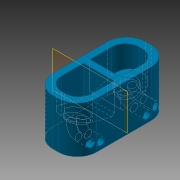
# Autodesk Inventor part: Line Tracker v3
Saved by Autodesk Inventor 2015 SP2 (Build 190223200, 223)
## iProperties
Created: 2015-04-19
Part Number: Line Tracker v3
Material: PLA Plastic
Document SubType Name: Modeling
Designer: Kyle
Density: 1 g/cm^3
Appearance: Carbon Fiber 1
Author: Kyle
Autodesk Inventor part; units mm, degrees
ref_plane "YZ Plane" through (0, 0, 0) normal (1, 0, 0) x (0, 1, 0)
ref_plane "XZ Plane" through (0, 0, 0) normal (0, 1, 0) x (-1, 0, 0)
sketch "Sketch1" plane through (0, 0, 0) normal (1, 0, 0) x (0, 1, 0)
  line L0 (0, 0) -> (0, 10.795)
  line L1 (0, 10.795) -> (10.795, 10.795)
  line L2 (10.795, 10.795) -> (10.795, 9.017)
  line L3 (10.795, 9.017) -> (5.8775, 9.017)
  line L4 (5.8775, 9.017) -> (3.81, 1.3008)
  line L5 (4.3488, 0.762) -> (10.795, 0.762)
  line L6 (10.795, 0.762) -> (10.795, 0)
  line L7 (0, 0) -> (10.795, 0) construction
  line L8 (3.81, 1.3008) -> (4.3488, 0.762)
  line L9 (0, 0) -> (0, -10.795)
  line L10 (0, -10.795) -> (10.795, -10.795)
  line L11 (10.795, -10.795) -> (10.795, -9.017)
  line L12 (10.795, -9.017) -> (5.8775, -9.017)
  line L13 (5.8775, -9.017) -> (3.81, -1.3008)
  line L14 (4.3488, -0.762) -> (10.795, -0.762)
  line L15 (10.795, -0.762) -> (10.795, 0)
  line L16 (3.81, -1.3008) -> (4.3488, -0.762)
  dimension "d0" = 10.795
  dimension "d1" = 105
  dimension "d8" = 0.762
  dimension "d33" = 3.81
  dimension "d34" = 10.795
  dimension "d35" = 0.762
  dimension "d36" = 1.778
  constraints: 34 end point, 7 symmetric about line, 4 perpendicular, 2 horizontal, 1 collinear, 1 vertical
  measures "d0" distance of L0.start L0.end
  measures "d1" angle of L4 L3
  measures "d8" distance of L5.end L6.end
  measures "d33" distance from line of L0 L4.end
  measures "d34" distance of L0.end L1.end
  measures "d35" distance of L4.end L5.start
  measures "d36" distance of L1.end L2.end
extrude "Extrusion1" add sketch "Sketch1" along normal mid plane 7.112
sketch "Sketch2" plane through (3.556, 0, 0) normal (1, 0, 0) x (0, 0, -1)
  line L0 (-10.795, 10.795) -> (10.795, 10.795)
  line L1 (10.795, 10.795) -> (10.795, 0)
  line L2 (10.795, 0) -> (-10.795, 0)
  line L3 (-10.795, 0) -> (-10.795, 10.795)
  point P0 (0, 0)
  constraints: 8 end point, 2 parallel, 1 coincident, 1 horizontal, 1 perpendicular
extrude "Extrusion2" add sketch "Sketch2" along normal blind 1.524
ref_plane "Work Plane1" through (0, 0, 0) normal (-1, 0, 0) x (0, 0, 1)
mirror "Mirror1" about plane through (0, 0, 0) normal (-1, 0, 0) of "Extrusion2"
ref_plane "Work Plane2" through (3.556, 5.8775, 0) normal (0, 0, 1) x (1, 0, 0)
sketch "Sketch3" plane through (-3.556, 3.81, -1.3008) normal (0, 0.9659258, 0.258819) x (1, 0, 0)
  circle A0 centre (3.556, 4.4884) radius 2.286
  line L0 (3.556, -2.2426) -> (3.556, 4.4884) construction
  line L1 (7.112, 1.2874) -> (0, 1.2874) construction
  dimension "d14" = 4.572
  dimension "d15" = 6.731
  constraints: 2 end point, 1 centre point, 1 perpendicular
  measures "d14" diameter of A0
  measures "d15" distance of L0.start L0.end
extrude "Extrusion3" cut sketch "Sketch3" against normal blind 1.016
mirror "Mirror2" about plane through (3.556, 5.8775, 0) normal (0, 0, 1) of "Extrusion3"
fillet "Fillet4" radius 3.175 4 edges at (3.556, 8.3363, -9.017) (-3.556, 8.3363, -9.017) (3.556, 8.3363, 9.017) (-3.556, 8.3363, 9.017)
fillet "Fillet5" radius 4.445 4 edges at (5.08, 5.3975, 10.795) (5.08, 5.3975, -10.795) (-5.08, 5.3975, -10.795) (-5.08, 5.3975, 10.795)
sketch "Sketch4" plane through (0, 3.9903, 5.8992) normal (0, 0.9659258, -0.258819) x (1, 0, 0)
  line L0 (0, 0.0029) -> (0, -1.1401) construction
  line L1 (0, 0.0029) -> (0, 1.1459) construction
  line L2 (0, 0.0029) -> (0, -1.1079) construction
  circle A0 centre (0, 1.1459) radius 0.8255
  circle A1 centre (0, -1.1401) radius 0.8255
  line L3 (2.1143, 0.0029) -> (2.1143, 2.2658) construction
  point P0 (0, 6.731)
  dimension "d43" = 1.143
  dimension "d44" = 1.651
  constraints: 8 end point, 3 vertical, 2 centre point, 2 coincident, 1 collinear, 1 equal radius, 1 point on line
  measures "d43" distance of L0.start L0.end
  measures "d44" diameter of A0
revolve "Revolution1" cut sketch "Sketch4" angle 90 about axis through (2.1143, 3.9896, 5.8964) along (0, 0.258819, 0.9659258)
mirror "Mirror3" about plane through (3.556, 5.8775, 0) normal (0, 0, 1) of "Revolution1"
sketch "Sketch6" plane through (2.1143, 4.7773, -7.6581) normal (-1, 0, 0) x (0, -1, 0)
  circle A0 centre (2.5341, 0.1105) radius 0.8255 projected
  circle A1 centre (2.5341, 0.1105) radius 0.8255
  circle A2 centre (3.1258, 2.3186) radius 0.8255 projected
  circle A3 centre (3.1258, 2.3186) radius 0.8255
  point P0 (4.7773, 7.6581)
  constraints: 2 centre point, 2 coincident, 2 concentric
extrude "Extrusion6" cut sketch "Sketch6" against normal up to next
mirror "Mirror10" about plane through (3.556, 5.8775, 0) normal (0, 0, 1) of "Extrusion6"
equation "\"d0\" = 0.5 * Base_Length"
equation "\"d1\" = Sensor_Angle"
equation "\"d33\" = Base_Thickness"
equation "\"d34\" = Mount_Height"
equation "\"d14\" = LED_Base"
equation "\"d15\" = Hole_to_Center"
equation "\"d18\" = Wire_Spacing"
equation "\"Wire_Spacing\" = 1.143"
equation "\"Wire_Diameter\" = 1.651"
equation "\"LED_Base\" = 4.572"
equation "\"Mount_Space\" = 16.51"
equation "\"Mount_Clearance\" = 3.175"
equation "\"Mount_Height\" = 10.795"
equation "\"Base_Length\" = 21.59"
equation "\"Base_Width\" = 10.16"
equation "\"Sensor_Angle\" = 105deg"
equation "\"Base_Thickness\" = 3.81"
equation "\"Hole_to_Center\" = 6.731"
equation "\"Tape_Width\" = 2.54"
body "Solid1"
